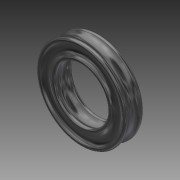
# Autodesk Inventor part: X-Ring 9.12x3.53
Saved by Autodesk Inventor 2019.4 (Build 234330000, 330)
## iProperties
Created: 2015-08-15
Part Number: X-Ring 9.12x3.53
Material: Gummi, Silikon
Document SubType Name: Modeling
Designer: rYan
Mass: 0.187427 g
Surface Area: 3.05947 cm^2
Volume: 0.149942 cm^3
Density: 1.25 g/cm^3
Appearance: Gummi - schwarz - Version 1.1
Author: rYan
Autodesk Inventor part; units mm, degrees
ref_plane "YZ Plane" through (0, 0, 0) normal (1, 0, 0) x (0, 1, 0)
ref_plane "XZ Plane" through (0, 0, 0) normal (0, 1, 0) x (-1, 0, 0)
ref_plane "XY Plane" through (0, 0, 0) normal (0, 0, 1) x (1, 0, 0)
sketch "Skizze1" plane through (0, 0, 0) normal (1, 0, 0) x (0, 1, 0)
  arc A0 (-1.0776, 8.2782) -> (-1.6567, 7.7263) centre (-1.365, 8) ccw
  arc A1 (-1.0776, 8.2782) -> (1.0776, 8.2782) centre (0, 9.3217) ccw
  arc A2 (1.6567, 7.7263) -> (1.0776, 8.2782) centre (1.365, 8) ccw
  arc A3 (1.6567, 7.7263) -> (1.6567, 5.6737) centre (2.7506, 6.7) ccw
  arc A4 (1.0776, 5.1218) -> (1.6567, 5.6737) centre (1.365, 5.4) ccw
  arc A5 (1.0776, 5.1218) -> (-1.0776, 5.1218) centre (0, 4.0783) ccw
  arc A6 (-1.6567, 5.6737) -> (-1.0776, 5.1218) centre (-1.365, 5.4) ccw
  arc A7 (-1.6567, 5.6737) -> (-1.6567, 7.7263) centre (-2.7506, 6.7) ccw
  line L0 (-1.365, 8) -> (1.365, 8) construction
  line L1 (1.365, 8) -> (1.365, 5.4) construction
  line L2 (1.365, 5.4) -> (-1.365, 5.4) construction
  line L3 (-1.365, 5.4) -> (-1.365, 8) construction
  line L4 (0, 11.186) -> (0, -1.8643) projected
  line L5 (-3.8509, 0) -> (3.8509, 0) construction
  line L6 (0, 8) -> (0, 5.4) construction
  line L7 (-1.365, 6.7) -> (1.365, 6.7) construction
  line L8 (-1.365, 8) -> (-1.765, 8) construction
  line L9 (-1.365, 5.4) -> (-1.765, 5.4) construction
  line L10 (-1.765, 5.4) -> (-1.765, 8) construction
  line L11 (-1.365, 8) -> (-1.365, 8.4) construction
  line L12 (-1.365, 5.4) -> (-1.365, 5) construction
  line L13 (1.365, 5.4) -> (1.365, 5) construction
  line L14 (-1.365, 5) -> (1.365, 5) construction
  line L15 (1.365, 8) -> (1.765, 8) construction
  line L16 (1.365, 5.4) -> (1.765, 5.4) construction
  line L17 (-1.365, 8.4) -> (1.365, 8.4) construction
  point P0 (0, 0)
  dimension "d0" = 3.4
  dimension "d1" = 10
  dimension "d2" = 3.53
  dimension "d3" = 1.5
  dimension "d4" = 0.4
  constraints: 32 end point, 25 point on circle, 10 tangent, 8 centre point, 7 parallel, 4 horizontal, 4 midpoint, 2 equal radius, 2 vertical, 1 point on line, 3 other
  measures "d0" distance of L12.end L11.end
  measures "d1" diameter of L14 L5
  measures "d2" distance of L8.end L15.end
  measures "d3" radius of A7
  measures "d4" radius of A0
revolve "Umdrehung1" add sketch "Skizze1" angle 360 about axis through (0, 0, 0) along (0, 1, 0)
